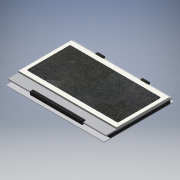
# Autodesk Inventor part: DisplayDummy
Saved by Autodesk Inventor 2017 (Build 210142000, 142)
## iProperties
Part Number: DisplayDummy
Material: Generisch
Document SubType Name: Modeling
Designer: aXe
Density: 1 g/cm^3
Appearance: Schwarz - Guss
Author: aXe
Autodesk Inventor part; units mm, degrees
ref_plane "YZ Plane" through (0, 0, 0) normal (1, 0, 0) x (0, 1, 0)
ref_plane "XZ Plane" through (0, 0, 0) normal (0, 1, 0) x (-1, 0, 0)
ref_plane "XY Plane" through (0, 0, 0) normal (0, 0, 1) x (1, 0, 0)
sketch "Skizze1" plane through (0, 0, 0) normal (0, 0, 1) x (1, 0, 0)
  line L0 (-47.05, -33.5) -> (47.05, -33.5)
  line L1 (47.05, -33.5) -> (47.05, 33.5)
  line L2 (47.05, 33.5) -> (-47.05, 33.5)
  line L3 (-47.05, 33.5) -> (-47.05, -33.5)
  line L4 (-47.05, -33.5) -> (47.05, 33.5) construction
  line L5 (47.05, -33.5) -> (-47.05, 33.5) construction
  point P0 (0, 0)
  dimension "d0" = 94.1
  dimension "d1" = 67
  constraints: 12 end point, 2 midpoint, 2 parallel, 1 horizontal, 1 perpendicular
  measures "d0" distance of L2.end L1.end
  measures "d1" distance of L1.end L0.end
extrude "LED_Platine" add sketch "Skizze1" along normal blind 0.55
sketch "Skizze2" plane through (0, 0, 0.55) normal (0, 0, 1) x (1, 0, 0)
  line L0 (47.05, 33.5) -> (-47.05, 33.5) projected
  line L1 (-47.05, 33.5) -> (-47.05, 30)
  line L2 (-47.05, 33.5) -> (-47.05, -33.5) projected
  line L3 (-47.05, -33.5) -> (47.05, -33.5) projected
  line L4 (47.05, -33.5) -> (47.05, -27.5)
  line L5 (47.05, -33.5) -> (47.05, 33.5) projected
  line L6 (-47.05, 30) -> (47.05, 30)
  line L7 (47.05, 30) -> (47.05, -27.5)
  line L8 (47.05, -27.5) -> (-47.05, -27.5)
  line L9 (-47.05, -27.5) -> (-47.05, 30)
  line L10 (-47.05, 30) -> (-45.75, 30)
  line L11 (-45.75, 30) -> (-45.75, 28.7)
  line L12 (-45.75, 28.7) -> (-47.05, 28.7)
  line L13 (-47.05, 28.7) -> (-47.05, 30)
  line L14 (47.05, -27.5) -> (45.75, -27.5)
  line L15 (45.75, -27.5) -> (45.75, -20.5)
  line L16 (45.75, -20.5) -> (47.05, -20.5)
  line L17 (47.05, -20.5) -> (47.05, -27.5)
  line L18 (-45.75, 28.7) -> (45.75, 28.7)
  line L19 (45.75, 28.7) -> (45.75, -20.5)
  line L20 (45.75, -20.5) -> (-45.75, -20.5)
  line L21 (-45.75, -20.5) -> (-45.75, 28.7)
  point P0 (0, 0)
  dimension "d4" = 3.5
  dimension "d5" = 6
  dimension "d8" = 1.3
  dimension "d9" = 1.3
  dimension "d10" = 1.3
  dimension "d11" = 7
  constraints: 36 end point, 8 parallel, 4 horizontal, 4 perpendicular, 2 point on line
  measures "d4" distance of L0.end L1.end
  measures "d5" distance of L3.end L4.end
  measures "d8" distance of L11.end L12.end
  measures "d9" distance of L10.end L11.end
  measures "d10" distance of L15.end L16.end
  measures "d11" distance of L14.end L15.end
extrude "LED_Rand" add sketch "Skizze2" along normal blind 3 separate body contours L5 L16 L19 L18 L11 L6 | L6 L11 L12 L2 | L5 L8 L15 L16 | L12 L21 L20 L15 L8 L2
sketch "Skizze3" plane through (0, 0, 0.55) normal (0, 0, 1) x (1, 0, 0)
  line L0 (45.75, -20.5) -> (-45.75, -20.5) projected
  line L1 (-45.75, -20.5) -> (-45.75, 28.7) projected
  line L2 (-45.75, 28.7) -> (45.75, 28.7) projected
  line L3 (45.75, 28.7) -> (45.75, -20.5) projected
  line L4 (-47.05, -27.5) -> (47.05, -27.5) projected
  line L5 (47.05, -27.5) -> (47.05, 30) projected
  line L6 (47.05, 30) -> (-47.05, 30) projected
  line L7 (-47.05, 30) -> (-47.05, -27.5) projected
  point P0 (0, 0)
extrude "LED_Beleuchtung" add sketch "Skizze3" along normal blind 3 separate body contours L0 L1 L2 L3
sketch "Skizze4" plane through (0, 0, 3.55) normal (0, 0, 1) x (1, 0, 0)
  line L0 (47.05, 30) -> (-47.05, 30) projected
  line L1 (-47.05, 30) -> (-47.05, -27.5) projected
  line L2 (47.05, -27.5) -> (47.05, 30) projected
  line L3 (-47.05, -27.5) -> (47.05, -27.5) projected
  line L4 (45.75, -20.5) -> (-45.75, -20.5) projected
  line L5 (-45.75, -20.5) -> (-47.05, -20.5)
  line L6 (-47.05, -20.5) -> (-47.05, -21.8)
  line L7 (-47.05, -21.8) -> (-45.75, -21.8)
  line L8 (-45.75, -21.8) -> (-45.75, -20.5)
  line L9 (-47.05, -21.8) -> (47.05, -21.8)
  line L10 (47.05, -21.8) -> (47.05, 30)
  line L11 (47.05, 30) -> (-47.05, 30)
  line L12 (-47.05, 30) -> (-47.05, -21.8)
  point P0 (0, 0)
  dimension "d16" = 1.3
  constraints: 16 end point, 4 parallel, 2 horizontal, 2 perpendicular, 1 point on line
  measures "d16" distance of L6.end L5.end
extrude "LCD_Back" add sketch "Skizze4" along normal blind 0.3 separate body contours L2 L9 L8 L5 L1 L0 | L5 L8 L7 L1
sketch "Skizze5" plane through (0, 0, 3.85) normal (0, 0, 1) x (1, 0, 0)
  line L0 (-47.05, -33.5) -> (47.05, -33.5) projected
  line L1 (47.05, -33.5) -> (47.05, 33.5) projected
  line L2 (47.05, 33.5) -> (-47.05, 33.5) projected
  line L3 (-47.05, 33.5) -> (-47.05, -33.5) projected
  line L4 (-47.05, 33.5) -> (-47.05, 31.55)
  line L5 (47.05, -33.5) -> (47.05, 33.5) projected
  line L6 (47.05, -33.5) -> (47.05, -31.55)
  line L7 (-47.05, 31.55) -> (47.05, 31.55)
  line L8 (47.05, 31.55) -> (47.05, -31.55)
  line L9 (47.05, -31.55) -> (-47.05, -31.55)
  line L10 (-47.05, -31.55) -> (-47.05, 31.55)
  point P0 (0, 0)
  dimension "d19" = 1.95
  dimension "d20" = 1.95
  constraints: 12 end point, 2 parallel, 2 point on line, 1 horizontal, 1 perpendicular
  measures "d19" distance of L2.end L4.end
  measures "d20" distance of L0.end L6.end
extrude "LCD_BackGlas" add sketch "Skizze5" along normal blind 1.15 separate body contours L3 L7 L1 L9
sketch "Skizze6" plane through (0, 0, 5) normal (0, 0, 1) x (1, 0, 0)
  line L0 (47.05, -31.55) -> (47.05, 31.55) projected
  line L1 (47.05, 31.55) -> (-47.05, 31.55) projected
  line L2 (-47.05, 31.55) -> (-47.05, -31.55) projected
  line L3 (-47.05, -31.55) -> (47.05, -31.55) projected
  line L4 (47.05, 31.55) -> (-47.05, 31.55) projected
  line L5 (-47.05, 31.55) -> (-47.05, 29.15)
  line L6 (-47.05, 30) -> (-47.05, -27.5) projected
  line L7 (47.05, -31.55) -> (47.05, 31.55) projected
  line L8 (47.05, -31.55) -> (47.05, -21.55)
  line L9 (-47.05, 29.15) -> (47.05, 29.15)
  line L10 (47.05, 29.15) -> (47.05, -21.55)
  line L11 (47.05, -21.55) -> (-47.05, -21.55)
  line L12 (-47.05, -21.55) -> (-47.05, 29.15)
  point P0 (0, 0)
  dimension "d23" = 2.4
  dimension "d24" = 10
  constraints: 12 end point, 2 parallel, 2 point on line, 1 horizontal, 1 perpendicular
  measures "d23" distance of L1.end L5.end
  measures "d24" distance of L0.start L8.end
extrude "LCD_FrontGlas" add sketch "Skizze6" along normal blind 1.5 separate body contours L11 L2 L9 L0
sketch "Skizze7" plane through (0, 0, 6.5) normal (0, 0, 1) x (1, 0, 0)
  line L0 (47.05, -21.55) -> (47.05, 29.15) projected
  line L1 (47.05, 29.15) -> (-47.05, 29.15) projected
  line L2 (-47.05, 29.15) -> (-47.05, -21.55) projected
  line L3 (-47.05, -21.55) -> (47.05, -21.55) projected
  line L4 (-47.05, 29.15) -> (-43.7, 29.15)
  line L5 (-43.7, 29.15) -> (-43.7, 24.6)
  line L6 (-43.7, 24.6) -> (-47.05, 24.6)
  line L7 (-47.05, 24.6) -> (-47.05, 29.15)
  line L8 (47.05, -21.55) -> (43.7, -21.55)
  line L9 (43.7, -21.55) -> (43.7, -17)
  line L10 (43.7, -17) -> (47.05, -17)
  line L11 (47.05, -17) -> (47.05, -21.55)
  line L12 (-42.7, 24.6) -> (42.7, 24.6)
  line L13 (43.7, 23.6) -> (43.7, -16)
  line L14 (42.7, -17) -> (-42.7, -17)
  line L15 (-43.7, -16) -> (-43.7, 23.6)
  arc A0 (-42.7, 24.6) -> (-43.7, 23.6) centre (-42.7, 23.6) ccw
  arc A1 (-43.7, -16) -> (-42.7, -17) centre (-42.7, -16) ccw
  arc A2 (42.7, -17) -> (43.7, -16) centre (42.7, -16) ccw
  arc A3 (43.7, 23.6) -> (42.7, 24.6) centre (42.7, 23.6) ccw
  point P0 (0, 0)
  dimension "d29" = 3.35
  dimension "d30" = 4.55
  dimension "d31" = 3.35
  dimension "d32" = 4.55
  dimension "d33" = 1
  constraints: 24 end point, 8 point on circle, 8 tangent, 6 parallel, 4 centre point, 4 point on line, 3 equal radius, 3 horizontal, 3 perpendicular
  measures "d29" distance of L5.end L6.end
  measures "d30" distance of L4.end L5.end
  measures "d31" distance of L9.end L10.end
  measures "d32" distance of L8.end L9.end
  measures "d33" radius of A0
extrude "LCD_AA" add sketch "Skizze7" along normal blind 0.1 separate body contours L12 A3 L13 A2 L14 A1 L15 A0
sketch "Skizze8" plane through (0, 0, 5) normal (0, 0, 1) x (1, 0, 0)
  line L0 (47.05, 31.55) -> (-47.05, 31.55) projected
  line L1 (47.05, -31.55) -> (47.05, 31.55) projected
  line L2 (47.05, 31.55) -> (-47.05, 31.55) projected
  line L3 (-47.05, 31.55) -> (-47.05, -31.55) projected
  line L4 (-47.05, -31.55) -> (47.05, -31.55) projected
  line L5 (-47.05, 31.55) -> (-25.05, 31.55)
  line L6 (-25.05, 31.55) -> (-18.05, 31.55)
  line L7 (-18.05, 31.55) -> (-18.05, 32.55)
  line L8 (-18.05, 32.55) -> (-25.05, 32.55)
  line L9 (-25.05, 32.55) -> (-25.05, 31.55)
  line L10 (-25.05, 31.55) -> (-18.05, 31.55)
  line L11 (-18.05, 31.55) -> (-18.05, 29.55)
  line L12 (-18.05, 29.55) -> (-25.05, 29.55)
  line L13 (-25.05, 29.55) -> (-25.05, 31.55)
  line L14 (47.05, 31.55) -> (25.05, 31.55)
  line L15 (25.05, 31.55) -> (18.05, 31.55)
  line L16 (18.05, 31.55) -> (18.05, 32.55)
  line L17 (18.05, 32.55) -> (25.05, 32.55)
  line L18 (25.05, 32.55) -> (25.05, 31.55)
  line L19 (18.05, 31.55) -> (25.05, 31.55)
  line L20 (25.05, 31.55) -> (25.05, 29.55)
  line L21 (25.05, 29.55) -> (18.05, 29.55)
  line L22 (18.05, 29.55) -> (18.05, 31.55)
  line L23 (-47.05, -31.55) -> (-25.05, -31.55)
  line L24 (-47.05, -31.55) -> (47.05, -31.55) projected
  line L25 (47.05, -31.55) -> (25.05, -31.55)
  line L26 (-25.05, -31.55) -> (25.05, -31.55)
  line L27 (25.05, -31.55) -> (25.05, -32.55)
  line L28 (25.05, -32.55) -> (-25.05, -32.55)
  line L29 (-25.05, -32.55) -> (-25.05, -31.55)
  line L30 (-25.05, -31.55) -> (25.05, -31.55)
  line L31 (25.05, -31.55) -> (25.05, -29.55)
  line L32 (25.05, -29.55) -> (-25.05, -29.55)
  line L33 (-25.05, -29.55) -> (-25.05, -31.55)
  point P0 (0, 0)
  dimension "d34" = 22
  dimension "d35" = 7
  dimension "d36" = 1
  dimension "d37" = 7
  dimension "d38" = 2
  dimension "d39" = 22
  dimension "d40" = 7
  dimension "d41" = 1
  dimension "d42" = 7
  dimension "d43" = 2
  dimension "d44" = 22
  dimension "d45" = 22
  dimension "d46" = 1
  dimension "d47" = 2
  constraints: 56 end point, 12 parallel, 6 horizontal, 6 perpendicular, 5 point on line
  measures "d34" distance of L2.end L5.end
  measures "d35" distance of L8.end L7.end
  measures "d36" distance of L7.end L6.end
  measures "d37" distance of L11.end L12.end
  measures "d38" distance of L10.end L11.end
  measures "d39" distance of L1.end L14.end
  measures "d40" distance of L16.end L17.end
  measures "d41" distance of L15.end L16.end
  measures "d42" distance of L20.end L21.end
  measures "d43" distance of L19.end L20.end
  measures "d44" distance of L3.end L23.end
  measures "d45" distance of L1.start L25.end
  measures "d46" distance of L26.end L27.end
  measures "d47" distance of L31.end L30.end
extrude "Extrusion9" add sketch "Skizze8" along normal blind 1 and the other way blind 2 separate body contours L20 L21 L22 L0 | L0 L16 L17 L18 | L27 L28 L29 L4 | L4 L33 L32 L31 | L11 L12 L13 L0 | L0 L9 L8 L7
